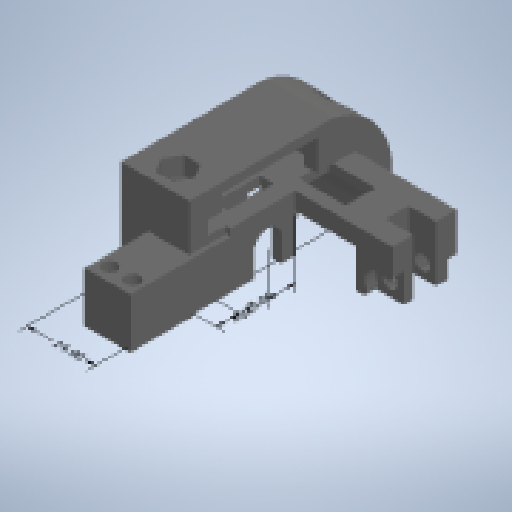
# Autodesk Inventor part: hand_motor_setter_base
Saved by Autodesk Inventor 2024.1 (Build 281209000, 209)
## iProperties
Created: 2025-01-23
Part Number: hand_motor_setter_base
Material: 一般
Document SubType Name: Modeling
Designer: hibik
Density: 1 g/cm^3
Appearance: 既定
Author: hibik
Autodesk Inventor part; units mm, degrees
ref_plane "YZ Plane" through (0, 0, 0) normal (1, 0, 0) x (0, 1, 0)
ref_plane "XZ Plane" through (0, 0, 0) normal (0, 1, 0) x (-1, 0, 0)
sketch "スケッチ1" plane through (0, 0, 0) normal (0, 1, 0) x (-1, 0, 0)
  line L0 (4.5, 6) -> (-4.5, 6) construction
  line L1 (-4.5, 6) -> (-4.5, -18) construction
  line L2 (-4.5, -18) -> (4.5, -18) construction
  line L3 (4.5, -18) -> (4.5, 6) construction
  line L4 (4.5, -6) -> (-4.5, -6)
  line L5 (0, -25.74) -> (0, 13.74) projected
  line L6 (0.5, -18) -> (0.5, -6) construction
  line L7 (4.6, -18.1) -> (-4.6, -18.1)
  line L8 (-4.6, -18.1) -> (-4.6, 6.1)
  line L9 (-4.6, 6.1) -> (4.6, 6.1)
  line L10 (4.6, 6.1) -> (4.6, -18.1)
  line L11 (0.4, -18.1) -> (0.4, -6)
  line L12 (-4.5, -6) -> (-4.6, -6)
  line L13 (4.5, -6) -> (4.6, -6)
  line L14 (6.6, -20.1) -> (-6.6, -20.1)
  line L15 (-6.6, -20.1) -> (-6.6, 8.1)
  line L16 (-6.6, 8.1) -> (6.6, 8.1)
  line L17 (6.6, 8.1) -> (6.6, -20.1)
  line L18 (0.4, -18.1) -> (-14.8, -18.1)
  line L19 (-14.8, -18.1) -> (-14.8, -6)
  line L20 (-14.8, -6) -> (0.4, -6)
  line L21 (0.4, -6) -> (0.4, -18.1)
  line L22 (-6.6, -20.1) -> (-14.8, -20.1)
  line L23 (-14.8, -20.1) -> (-14.8, -18.1)
  point P0 (0, 0)
  point P1 (0, -6)
  point P2 (-6.6, -6)
  point P3 (0, -20.1)
  point P4 (-6.6, -6)
  dimension "d0" = 6
  dimension "d1" = 12
  dimension "d2" = 12
  dimension "d3" = 9
  dimension "d4" = 4
  dimension "d5" = 0.1
  dimension "d6" = 0.1
  dimension "d7" = 0.1
  dimension "d8" = 0.1
  dimension "d9" = 0.1
  dimension "d10" = 2
  dimension "d11" = 2
  dimension "d12" = 15.2
  constraints: 46 end point, 8 parallel, 7 midpoint, 7 perpendicular, 6 horizontal, 4 point on line, 1 collinear, 1 horizontal alignment, 1 vertical alignment, 1 other
  measures "d0" distance from line of L0 point (0, 0)
  measures "d1" distance between parallel lines of L0 L4
  measures "d2" distance between parallel lines of L2 L4
  measures "d3" distance of L1.end L2.end
  measures "d4" distance between parallel lines of L3 L6
  measures "d5" distance between parallel lines of L8 L1
  measures "d6" distance between parallel lines of L10 L3
  measures "d7" distance between parallel lines of L7 L2
  measures "d8" distance between parallel lines of L9 L0
  measures "d9" distance between parallel lines of L11 L6
  measures "d10" distance between parallel lines of L15 L8
  measures "d11" distance between parallel lines of L14 L7
  measures "d12" distance of L19.end L20.end
extrude "押し出し1" add sketch "スケッチ1" against normal blind 2
extrude "押し出し2" add sketch "スケッチ1" against normal blind 12.2 contours L13 L10 L7 L11 L4 | L11 L7 L5 L4 | L10 L9 L5 L16 L17 L14 L7 | L5 L7 L8 L12 L4 | L5 L14 L15 L18 L7 | L9 L8 L20 L15 L16 L5 | L8 L18 L15 L20 | L15 L18 L19 L20 | L22 L23 L18 L15
sketch "スケッチ2" plane through (14.8, 0, -6) normal (1, 0, 0) x (0, 0, -1)
  line L0 (0, 0) -> (0, -12.2) projected
  line L1 (0, -2) -> (14.1, -2)
  line L2 (14.1, 0) -> (14.1, -12.2) projected
  line L3 (0, 0) -> (14.1, 0) projected
  circle A0 centre (6.05, -7.1) radius 6.05
  line L4 (0, 0) -> (0, -12.2) projected
  line L5 (0, 0) -> (14.1, 0) projected
  line L6 (0, 0) -> (0, -12.2) projected
  line L7 (14.1, -12.2) -> (0, -12.2) projected
  line L8 (14.1, 0) -> (14.1, -12.2) projected
  line L9 (12.1, 0) -> (12.1, -12.2)
  point P0 (-6, 0)
  point P1 (14.1, -7.1)
  point P2 (9.3046, -2)
  point P3 (2.7954, -2)
  point P4 (0, -7.1)
  point P5 (2.7954, -12.2)
  point P6 (9.3046, -12.2)
  point P7 (0, -7.1)
  point P8 (12.1, -7.1)
  dimension "d17" = 2
  dimension "d18" = 5.1
  dimension "d21" = 2
  constraints: 4 end point, 4 point on line, 2 tangent, 1 centre point, 1 horizontal, 1 perpendicular
  measures "d17" distance between parallel lines of L3 L1
  measures "d18" distance from line of L1 A0.centre
  measures "d21" distance between parallel lines of L2 L9
extrude "押し出し3" cut sketch "スケッチ2" against normal blind 15.2 contours A0 L7 L0 | A0 L1 L7 | L9 L7 A0
sketch "スケッチ3" plane through (6.6, 0, 8.1) normal (1, 0, 0) x (0, 0, -1)
  circle A0 centre (8.1, -7.1) radius 3
  line L0 (14.1, -12.2) -> (0, -12.2) projected
  line L1 (5.1, -12.2) -> (11.1, -12.2)
  line L2 (11.1, -12.2) -> (11.1, -7.1)
  line L3 (11.1, -7.1) -> (5.1, -7.1)
  line L4 (5.1, -7.1) -> (5.1, -12.2)
  point P0 (8.1, 0)
  dimension "d22" = 6
  dimension "d23" = 7.1
  constraints: 8 end point, 2 parallel, 2 vertical, 1 horizontal, 1 perpendicular, 1 point on line, 1 vertical alignment, 3 other
  measures "d23" distance of point (8.1, 0) point (8.1, -7.1)
extrude "押し出し4" cut sketch "スケッチ3" against normal up to surface (2 mm away)
fillet "フィレット1" radius 0.5 2 edges at (10.7, -7.1, -6) (2.1, -7.1, -6)
sketch "スケッチ4" plane through (-0.4, 0, -6) normal (1, 0, 0) x (0, 0, -1)
  line L0 (-14.1, -12.2) -> (14.1, -12.2) projected
  line L1 (0, -12.2) -> (12.1, -12.2)
  line L2 (12.1, -12.2) -> (12.1, -2)
  line L3 (12.1, -2) -> (0, -2)
  line L4 (0, -2) -> (0, -12.2)
  line L5 (12.1, -7.1) -> (12.1, -12.2) projected
  line L6 (2.7954, -2) -> (9.3046, -2) projected
  point P0 (-6, 0)
  constraints: 8 end point, 2 collinear, 2 parallel, 1 horizontal, 1 midpoint, 1 perpendicular
extrude "押し出し5" cut sketch "スケッチ4" against normal up to surface (4.2 mm away)
ref_plane "作業平面1" through (-3.6, -12.2, 6.1) normal (1, 0, 0) x (0, 0, -1)
sketch "スケッチ5" plane through (-3.6, -12.2, 6.1) normal (1, 0, 0) x (0, 0, -1)
  line L0 (0, 10.2) -> (7.1, 10.2)
  line L1 (7.1, 10.2) -> (7.1, 5.2)
  line L2 (7.1, 5.2) -> (0, 5.2)
  line L3 (0, 5.2) -> (0, 10.2)
  line L4 (9.1, 0) -> (9.1, 5.1) projected
  point P0 (6.1, 12.2)
  dimension "d30" = 5
  dimension "d34" = 2
  constraints: 8 end point, 2 parallel, 1 horizontal, 1 perpendicular
  measures "d30" distance of L0.end L1.end
  measures "d34" distance between parallel lines of L1 L4
extrude "押し出し6" add sketch "スケッチ5" along normal blind 1.5
fillet "フィレット2" radius 3 2 edges at (-2.85, -7, -1) (-2.85, -7, 6.1)
sketch "スケッチ6" plane through (0, 0, 0) normal (0, 1, 0) x (1, 0, 0)
  line L0 (-6.6, -8.1) -> (6.6, -8.1) projected
  line L1 (5.6, -8.1) -> (2.6, -8.1)
  line L2 (2.6, -8.1) -> (2.6, -0.1)
  line L3 (2.6, -0.1) -> (5.6, -0.1)
  line L4 (5.6, -0.1) -> (5.6, -8.1)
  line L5 (6.6, -8.1) -> (6.6, 6) projected
  line L6 (-9.3, -8.1) -> (-7.3, -8.1)
  line L7 (-7.3, -8.1) -> (-7.3, 13.8)
  line L8 (-7.3, 13.8) -> (-9.3, 13.8)
  line L9 (-9.3, 13.8) -> (-9.3, -8.1)
  line L10 (-4.6, -6.1) -> (4.6, -6.1) projected
  line L11 (-7.3, -8.1) -> (2.6, -8.1)
  line L12 (2.6, -8.1) -> (2.6, -6.1)
  line L13 (2.6, -6.1) -> (-7.3, -6.1)
  line L14 (-7.3, -6.1) -> (-7.3, -8.1)
  line L15 (-9.3, 13.8) -> (2.9, 13.8)
  line L16 (2.9, 13.8) -> (2.9, 15.8)
  line L17 (2.9, 15.8) -> (-9.3, 15.8)
  line L18 (-9.3, 15.8) -> (-9.3, 13.8)
  line L19 (-9.3, 12.3) -> (-7.3, 12.3)
  line L20 (-9.3, -4.6) -> (-7.3, -4.6)
  line L21 (-7.3, -1.4667) -> (-9.3, -1.4667)
  line L22 (-9.3, -1.4667) -> (-9.3, 1.5333)
  line L23 (-9.3, 1.5333) -> (-7.3, 1.5333)
  line L24 (-7.3, 1.5333) -> (-7.3, -1.4667)
  line L25 (-7.3, 6.1667) -> (-9.3, 6.1667)
  line L26 (-9.3, 6.1667) -> (-9.3, 9.1667)
  line L27 (-9.3, 9.1667) -> (-7.3, 9.1667)
  line L28 (-7.3, 9.1667) -> (-7.3, 6.1667)
  circle A0 centre (-4.5, 8.6) radius 1
  circle A1 centre (-4.5, -0.9) radius 1
  line L29 (-9.3, 3.85) -> (-0.8107, 3.85)
  line L30 (2.9, 15.8) -> (-9.3, 15.8)
  line L31 (-9.3, 15.8) -> (-9.3, 20.1)
  line L32 (-9.3, 20.1) -> (2.9, 20.1)
  line L33 (2.9, 20.1) -> (2.9, 15.8)
  line L34 (14.8, 20.1) -> (-6.6, 20.1) projected
  point P0 (0, 0)
  point P1 (-9.3, 6.1667)
  point P2 (-7.3, 3.85)
  point P3 (2.6, -8.1)
  point P4 (2.6, -8.1)
  dimension "d35" = 4
  dimension "d36" = 8
  dimension "d37" = 3
  dimension "d40" = 9.9
  dimension "d41" = 2
  dimension "d42" = 19.9
  dimension "d43" = 2
  dimension "d44" = 10.2
  dimension "d45" = 1.5
  dimension "d46" = 1.5
  dimension "d53" = 3
  dimension "d54" = 3
  dimension "d55" = 4.6333
  dimension "d56" = 4.6333
  dimension "d57" = 4.6333
  dimension "d60" = 2
  dimension "d61" = 2
  dimension "d62" = 7.1
  dimension "d63" = 9.5
  constraints: 62 end point, 14 parallel, 12 point on line, 9 perpendicular, 8 horizontal, 3 collinear, 2 centre point, 1 symmetric about line, 1 vertical alignment, 1 other
  measures "d35" distance between parallel lines of L5 L2
  measures "d36" distance of L3.end L1.start
  measures "d37" distance between parallel lines of L4 L2
  measures "d40" distance between parallel lines of L2 L7
  measures "d41" distance of L6.start L6.end
  measures "d42" distance between parallel lines of L8 L13
  measures "d43" distance of L17.end L8.end
  measures "d44" distance between parallel lines of L16 L7
  measures "d45" distance between parallel lines of L15 L19
  measures "d46" distance between parallel lines of L13 L20
  measures "d53" distance between parallel lines of L21 L23
  measures "d54" distance between parallel lines of L27 L25
  measures "d55" distance between parallel lines of L13 L21
  measures "d56" distance between parallel lines of L25 L23
  measures "d57" distance between parallel lines of L15 L27
  measures "d60" diameter of A0
  measures "d61" diameter of A1
  measures "d62" distance from line of L2 A1.centre
  measures "d63" distance of A1.centre A0.centre
extrude "押し出し7" add sketch "スケッチ6" along normal blind 6.6 contours L11 L7 L13 L10 L2 L0 | L2 L3 L4 L0 | L6 L9 L20 L7 | L9 L23 L7 L21 | L9 L27 L7 L25 | L9 L8 L7 L19 | L18 L17 L16 L15 L8 | L31 L32 L33 L17 | A0 | A1
chamfer "面取り1" distance 6 distance2 2 1 edges at (5.6, 3.3, 0.1) measured on face at (5.6, 2.2, 5.4333)
sketch "スケッチ7" plane through (-6.6, -12.2, -20.1) normal (-1, 0, 0) x (0, 0, 1)
  line L0 (0, 12.2) -> (0, 0) projected
  line L1 (28.2, 0) -> (0, 0) projected
  line L2 (28.2, 12.2) -> (28.2, 0) projected
  line L3 (26.2, 12.2) -> (28.2, 12.2) projected
  line L4 (6.3, 12.2) -> (26.2, 12.2) projected
  line L5 (0, 12.2) -> (6.3, 12.2) projected
  point P0 (20.1, 12.2)
extrude "押し出し8" add sketch "スケッチ7" along normal up to surface (2.7 mm away)
sketch "スケッチ8" plane through (0, 6.6, 0) normal (0, 1, 0) x (1, 0, 0)
  line L0 (14.8, 20.1) -> (-9.3, 20.1) projected
  line L1 (-9.3, -8.1) -> (5.6, -8.1)
  line L2 (5.6, -8.1) -> (5.6, 20.1)
  line L3 (5.6, 20.1) -> (-9.3, 20.1)
  line L4 (-9.3, 20.1) -> (-9.3, -8.1)
  line L5 (5.6, -8.1) -> (5.6, -6.1) projected
  circle A0 centre (-1.85, 23.1) radius 1.6
  circle A1 centre (-1.85, -11.1) radius 1.6
  line L6 (5.6, 6) -> (-9.3, 6)
  line L7 (-9.3, -8.1) -> (5.6, -8.1)
  line L8 (5.6, -8.1) -> (5.6, -16.1)
  line L9 (5.6, -16.1) -> (-9.3, -16.1)
  line L10 (-9.3, -16.1) -> (-9.3, -8.1)
  line L11 (-9.3, 20.1) -> (5.6, 20.1)
  line L12 (5.6, 20.1) -> (5.6, 28.1)
  line L13 (5.6, 28.1) -> (-9.3, 28.1)
  line L14 (-9.3, 28.1) -> (-9.3, 20.1)
  line L15 (-9.3, 20.1) -> (-9.3, -8.1) projected
  line L16 (-9.3, -8.1) -> (5.6, -8.1) projected
  point P0 (0, 0)
  point P1 (-1.85, 20.1)
  dimension "d64" = 3.2
  dimension "d65" = 3.2
  dimension "d66" = 3
  dimension "d67" = 8
  constraints: 26 end point, 6 parallel, 5 collinear, 3 horizontal, 3 midpoint, 3 perpendicular, 2 centre point, 2 vertical alignment, 1 point on line, 1 symmetric about line, 1 other
  measures "d64" diameter of A0
  measures "d65" diameter of A1
  measures "d66" distance from line of A0.centre L0
  measures "d67" distance of L13.end L3.end
extrude "押し出し9" add sketch "スケッチ8" along normal blind 2
extrude "押し出し10" add sketch "スケッチ8" against normal up to surface (18.8 mm away) contours L0 L14 L13 L12 | L1 L8 L9 L10
sketch "スケッチ9" plane through (0, 8.6, 0) normal (0, 1, 0) x (1, 0, 0)
  circle A0 centre (-1.85, -11.1) radius 1.6 projected
  circle A1 centre (-1.85, 23.1) radius 1.6 projected
  line L0 (1.4409, -11.1) -> (-0.2046, -13.95)
  line L1 (-0.2046, -13.95) -> (-3.4954, -13.95)
  line L2 (-3.4954, -13.95) -> (-5.1409, -11.1)
  line L3 (-5.1409, -11.1) -> (-3.4954, -8.25)
  line L4 (-3.4954, -8.25) -> (-0.2046, -8.25)
  line L5 (-0.2046, -8.25) -> (1.4409, -11.1)
  line L6 (-0.2046, 25.95) -> (1.4409, 23.1)
  line L7 (1.4409, 23.1) -> (-0.2046, 20.25)
  line L8 (-0.2046, 20.25) -> (-3.4954, 20.25)
  line L9 (-3.4954, 20.25) -> (-5.1409, 23.1)
  line L10 (-5.1409, 23.1) -> (-3.4954, 25.95)
  line L11 (-3.4954, 25.95) -> (-0.2046, 25.95)
  point P0 (0, 0)
  dimension "d72" = 5.7
  constraints: 24 end point, 2 coincident, 2 horizontal, 1 parallel, 26 other
  measures "d72" distance between parallel lines of L1 L4
extrude "押し出し11" cut sketch "スケッチ9" against normal blind 6.5 contours A0 | A1 | L0 L1 L2 L3 L4 L5 | L6 L7 L8 L9 L10 L11
sketch "スケッチ10" plane through (0, 8.6, 0) normal (0, 1, 0) x (1, 0, 0)
  circle A0 centre (-1.85, -11.1) radius 1.6 projected
  circle A1 centre (-1.85, 23.1) radius 1.6 projected
  line L0 (-3.6398, -8) -> (-0.0602, -8)
  line L1 (-0.0602, -8) -> (1.7296, -11.1)
  line L2 (1.7296, -11.1) -> (-0.0602, -14.2)
  line L3 (-0.0602, -14.2) -> (-3.6398, -14.2)
  line L4 (-3.6398, -14.2) -> (-5.4296, -11.1)
  line L5 (-5.4296, -11.1) -> (-3.6398, -8)
  line L6 (-3.6398, 26.2) -> (-0.0602, 26.2)
  line L7 (-0.0602, 26.2) -> (1.7296, 23.1)
  line L8 (1.7296, 23.1) -> (-0.0602, 20)
  line L9 (-0.0602, 20) -> (-3.6398, 20)
  line L10 (-3.6398, 20) -> (-5.4296, 23.1)
  line L11 (-5.4296, 23.1) -> (-3.6398, 26.2)
  line L12 (-0.2046, -13.95) -> (-3.4954, -13.95) projected
  line L13 (-0.2046, 20.25) -> (-3.4954, 20.25) projected
  point P0 (0, 0)
  dimension "d75" = 6.2
  constraints: 24 end point, 2 coincident, 2 parallel, 1 equal length, 26 other
  measures "d75" distance between parallel lines of L0 L3
extrude "押し出し12" cut sketch "スケッチ10" against normal blind 4 contours A0 | A1 | L0 L1 L2 L3 L4 L5 | L6 L7 L8 L9 L10 L11
sketch "スケッチ11" plane through (14.8, 0, -6) normal (1, 0, 0) x (0, 0, -1)
  arc A0 (0, -3.6215) -> (0.9237, -3.887) centre (0.5, -3.6215) ccw projected
  arc A1 (2.7954, -2) -> (0.9237, -3.887) centre (6.05, -7.1) ccw projected
  line L0 (2.7954, -2) -> (9.3046, -2) projected
  arc A2 (12.1, -7.1) -> (9.3046, -2) centre (6.05, -7.1) ccw projected
  line L1 (12.1, -7.1) -> (12.1, -12.2) projected
  line L2 (14.1, -12.2) -> (12.1, -12.2) projected
  line L3 (14.1, 0) -> (14.1, -12.2) projected
  line L4 (0, 0) -> (14.1, 0) projected
  line L5 (0, 0) -> (0, -3.6215) projected
  line L6 (9.3046, -2) -> (14.1, -2)
  point P0 (-6, 0)
  constraints: 2 end point, 1 perpendicular, 1 point on line
extrude "押し出し13" add sketch "スケッチ11" along normal blind 5 contours L5 L4 L3 L6 L0 A1 A0
sketch "スケッチ12" plane through (19.8, 0, -6) normal (1, 0, 0) x (0, 0, -1)
  line L0 (0, -7.1) -> (0, -12.2) projected
  line L1 (14.1, 0) -> (0, 0) projected
  line L2 (14.1, -2) -> (14.1, -12.2) projected
  line L3 (14.1, -12.2) -> (0, -12.2)
  line L4 (0, -12.2) -> (0, 0)
  line L5 (0, 0) -> (14.1, 0)
  line L6 (14.1, 0) -> (14.1, -12.2)
  point P0 (-6, 0)
  constraints: 8 end point, 2 parallel, 1 horizontal, 1 perpendicular
extrude "押し出し14" add sketch "スケッチ12" along normal blind 2
sketch "スケッチ13" plane through (14.8, -12.2, -20.1) normal (0, 0, -1) x (-1, 0, 0)
  line L0 (8.2, 12.2) -> (-7, 12.2) projected
  line L1 (-7, 12.2) -> (-13, 12.2)
  line L2 (-13, 12.2) -> (-13, 0)
  line L3 (-13, 0) -> (-7, 0)
  line L4 (-7, 0) -> (-7, 12.2)
  circle A0 centre (-10, 3) radius 1.6
  line L5 (-5, 0) -> (-7, 0) projected
  point P0 (14.8, 12.2)
  dimension "d98" = 3.2
  dimension "d99" = 3
  dimension "d100" = 3
  dimension "d101" = 6
  constraints: 8 end point, 2 parallel, 1 centre point, 1 collinear, 1 horizontal, 1 perpendicular
  measures "d98" diameter of A0
  measures "d99" distance from line of L3 A0.centre
  measures "d100" distance from line of L2 A0.centre
  measures "d101" distance of L0.end L1.end
extrude "押し出し15" add sketch "スケッチ13" against normal up to surface (14.1 mm away)
sketch "スケッチ14" plane through (19.8, -12.2, -20.1) normal (0, -1, 0) x (1, 0, 0)
  line L0 (8, 0) -> (8, 14.1) projected
  line L1 (8, 4.55) -> (2, 4.55)
  line L2 (2, 4.55) -> (2, 9.55)
  line L3 (2, 9.55) -> (8, 9.55)
  line L4 (8, 9.55) -> (8, 4.55)
  line L5 (0, 14.1) -> (0, 0) projected
  point P0 (-19.8, 20.1)
  point P1 (2, 7.05)
  point P2 (0, 7.05)
  point P3 (8, 9.55)
  dimension "d104" = 2
  dimension "d105" = 5
  constraints: 8 end point, 2 midpoint, 2 parallel, 1 horizontal, 1 horizontal alignment, 1 perpendicular, 1 point on line
  measures "d104" distance between parallel lines of L5 L2
  measures "d105" distance of L1.end L2.end
extrude "押し出し16" cut sketch "スケッチ14" against normal through all
sketch "スケッチ15" plane through (14.8, -12.2, -20.1) normal (0, 0, -1) x (-1, 0, 0)
  circle A0 centre (-10, 3) radius 1.6 projected
  line L0 (-11.7321, 0) -> (-13.4641, 3)
  line L1 (-13.4641, 3) -> (-11.7321, 6)
  line L2 (-11.7321, 6) -> (-8.2679, 6)
  line L3 (-8.2679, 6) -> (-6.5359, 3)
  line L4 (-6.5359, 3) -> (-8.2679, 0)
  line L5 (-8.2679, 0) -> (-11.7321, 0)
  line L6 (-5, 0) -> (-13, 0) projected
  line L7 (-13, 12.2) -> (-13, 0) projected
  point P0 (14.8, 12.2)
  point P1 (-13, 3.8038)
  point P2 (-11.7321, 0)
  constraints: 12 end point, 1 coincident, 1 collinear, 1 horizontal, 13 other
extrude "押し出し17" cut sketch "スケッチ15" against normal blind 2 contours A0 | L6 L7 L0 | L0 L7 L1 L2 L3 L4 L5
sketch "スケッチ16" plane through (6.6, -3.6215, -6) normal (0, 0, 1) x (1, 0, 0)
  circle A0 centre (18.2, -5.5785) radius 1.6 projected
  circle A1 centre (18.2, -5.5785) radius 3
  circle A2 centre (18.2, -5.5785) radius 1.6 projected
  line L0 (13.2, 0) -> (0, 0) projected
  line L1 (13.2, 0) -> (13.2, -8.5785) projected
  line L2 (13.2, -8.5785) -> (21.2, -8.5785) projected
  line L3 (21.2, 3.6215) -> (21.2, -8.5785) projected
  line L4 (0, 3.6215) -> (21.2, 3.6215) projected
  line L5 (0, 3.6215) -> (0, 0) projected
  point P0 (-6.6, 3.6215)
  point P1 (21.2, -5.5785)
  point P2 (18.2, -8.5785)
  constraints: 1 centre point, 1 coincident, 1 tangent
extrude "押し出し18" cut sketch "スケッチ16" against normal blind 2.5 contours A1 | L3 L2 A1
fillet "フィレット3" radius 1 2 edges at (24.8, -12.2, -7.25) (27.8, -9.2, -7.25)
sketch "スケッチ17" plane through (0, 0, 0) normal (0, 1, 0) x (1, 0, 0)
  circle A0 centre (-4.5, 8.6) radius 1 projected
  circle A1 centre (-4.5, -0.9) radius 1 projected
  line L0 (27.8, 10.55) -> (21.8, 10.55) projected
  line L1 (21.8, 10.55) -> (21.8, 15.55) projected
  line L2 (21.8, 15.55) -> (27.8, 15.55) projected
  line L3 (27.8, 20.1) -> (27.8, 15.55) projected
  line L4 (27.8, 20.1) -> (5.6, 20.1) projected
  line L5 (5.6, 20.1) -> (2.9, 20.1) projected
  line L6 (-7.3, 13.8) -> (2.9, 13.8) projected
  line L7 (-7.3, 12.3) -> (-7.3, 13.8) projected
  line L8 (-7.3, -6.1) -> (2.6, -6.1) projected
  line L9 (2.6, -6.1) -> (2.6, -0.1) projected
  line L10 (2.6, -0.1) -> (3.6, -0.1) projected
  line L11 (5.6, -6.1) -> (3.6, -0.1) projected
  line L12 (5.6, -6.1) -> (5.6, -8.1) projected
  line L13 (5.6, -8.1) -> (6.6, -8.1) projected
  line L14 (6.6, -8.1) -> (6.6, 6) projected
  line L15 (6.6, 6) -> (27.8, 6) projected
  line L16 (27.8, 10.55) -> (27.8, 6) projected
  line L17 (2.6, -6.1) -> (2.6, -0.1) projected
  line L18 (2.6, -0.1) -> (6.6, -0.1)
  line L19 (6.6, -0.1) -> (6.6, -12.1)
  line L20 (6.6, -12.1) -> (2.6, -12.1)
  line L21 (2.6, -12.1) -> (2.6, -0.1)
  line L22 (6.6, -8.1) -> (6.6, 6) projected
  line L23 (2.9, 20.1) -> (2.9, 13.8) projected
  line L24 (-9.3, 12.3) -> (-7.3, 12.3) projected
  line L25 (-9.3, 12.3) -> (-9.3, 9.1667) projected
  line L26 (-7.3, 9.1667) -> (-9.3, 9.1667) projected
  line L27 (-7.3, 6.1667) -> (-7.3, 9.1667) projected
  line L28 (-9.3, 6.1667) -> (-7.3, 6.1667) projected
  line L29 (-9.3, 6.1667) -> (-9.3, 1.5333) projected
  line L30 (-7.3, 1.5333) -> (-9.3, 1.5333) projected
  line L31 (-7.3, -1.4667) -> (-7.3, 1.5333) projected
  line L32 (-9.3, -1.4667) -> (-7.3, -1.4667) projected
  line L33 (-9.3, -1.4667) -> (-9.3, -4.6) projected
  line L34 (-7.3, -4.6) -> (-9.3, -4.6) projected
  line L35 (-7.3, -6.1) -> (-7.3, -4.6) projected
  point P0 (0, 0)
  dimension "d116" = 12
  constraints: 8 end point, 2 parallel, 1 collinear, 1 horizontal, 1 perpendicular
  measures "d116" distance of L18.end L19.end
extrude "押し出し19" cut sketch "スケッチ17" along normal up to surface (6.6 mm away) contours L14 L13 L12 L11 L18 | L19 L20 L21 L9 L10 L11 L12 L13
sketch "スケッチ18" plane through (0, 0, 0) normal (0, 1, 0) x (1, 0, 0)
  line L0 (2.9, 11.8) -> (5.6, 11.8)
  line L1 (5.6, 11.8) -> (5.6, 20.1)
  line L2 (5.6, 20.1) -> (2.9, 20.1)
  line L3 (2.9, 20.1) -> (2.9, 11.8)
  line L4 (5.6, 20.1) -> (2.9, 20.1) projected
  line L5 (5.6, -12.1) -> (5.6, 20.1) projected
  line L6 (2.9, 20.1) -> (2.9, 13.8) projected
  line L7 (-7.3, 13.8) -> (2.9, 13.8) projected
  point P0 (0, 0)
  dimension "d122" = 2
  constraints: 8 end point, 3 collinear, 2 parallel, 1 horizontal, 1 perpendicular
  measures "d122" distance between parallel lines of L7 L0
extrude "押し出し20" add sketch "スケッチ18" along normal up to surface (6.6 mm away)
sketch "スケッチ23" plane through (6.6, 0, 8.1) normal (1, 0, 0) x (0, 0, -1)
  line L0 (11.1, -7.1) -> (11.1, -12.2) projected
  line L1 (14.1, -12.2) -> (11.1, -12.2) projected
  line L2 (14.1, -7.1) -> (14.1, -12.2) projected
  arc A0 (15.0237, -3.887) -> (14.1, -7.1) centre (20.15, -7.1) ccw projected
  arc A1 (14.1, -3.6215) -> (15.0237, -3.887) centre (14.6, -3.6215) ccw projected
  line L3 (14.1, 0) -> (14.1, -3.6215) projected
  line L4 (0, 0) -> (14.1, 0) projected
  line L5 (0, 0) -> (0, -12.2) projected
  line L6 (5.1, -12.2) -> (0, -12.2) projected
  line L7 (5.1, -12.2) -> (5.1, -7.1) projected
  arc A2 (11.1, -7.1) -> (5.1, -7.1) centre (8.1, -7.1) ccw projected
  arc A3 (11.1, -7.1) -> (5.1, -7.1) centre (8.1, -7.1) ccw projected
  circle A4 centre (8.1, -7.1) radius 5.5
  line L8 (8.1, -1.6) -> (-21.9, -1.6)
  line L9 (-21.9, -1.6) -> (-21.9, -12.6)
  line L10 (-21.9, -12.6) -> (8.1, -12.6)
  line L11 (8.1, -12.6) -> (8.1, -1.6)
  line L12 (-8, 8.6) -> (-8, -12.2) projected
  line L13 (-8, -12.2) -> (-8, -12.6)
  line L14 (11.1, -12.2) -> (11.1, -7.1) projected
  arc A5 (11.1, -7.1) -> (5.1, -7.1) centre (8.1, -7.1) ccw projected
  line L15 (5.1, -7.1) -> (5.1, -12.2) projected
  line L16 (2, -12.2) -> (5.1, -12.2) projected
  line L17 (2, -2) -> (2, -12.2) projected
  line L18 (14.1, -2) -> (2, -2) projected
  line L19 (14.1, -2) -> (14.1, -3.6215) projected
  arc A6 (14.1, -3.6215) -> (15.0237, -3.887) centre (14.6, -3.6215) ccw projected
  arc A7 (15.0237, -3.887) -> (14.1, -7.1) centre (20.15, -7.1) ccw projected
  line L20 (14.1, -7.1) -> (14.1, -12.2) projected
  line L21 (11.1, -12.2) -> (14.1, -12.2) projected
  line L22 (2, -2) -> (2, -12.2) projected
  line L23 (2, -12.2) -> (2, -12.6)
  line L24 (2, -2) -> (2, -1.6)
  line L25 (-8, -12.2) -> (0, -12.2) projected
  point P0 (8.1, 0)
  dimension "d138" = 11
  dimension "d139" = 30
  constraints: 14 end point, 3 horizontal, 3 perpendicular, 3 point on line, 2 parallel, 1 coincident, 1 collinear, 1 vertical alignment, 2 other
  measures "d139" distance of L9.end L10.end
extrude "押し出し24" add sketch "スケッチ23" against normal blind 10 contours L10 L9 L8 L12 L13 | L6 L5 L8 L24 L17 | L12 L8 L5 L25
sketch "スケッチ24" plane through (0, -2, 0) normal (0, -1, 0) x (1, 0, 0)
  line L0 (2.9, 5.1) -> (-0.1, 5.1)
  line L1 (-0.1, 5.1) -> (-0.1, -5)
  line L2 (-0.1, -5) -> (2.9, -5)
  line L3 (4.6, -3) -> (4.6, 3) projected
  line L4 (-4.6, 6.1) -> (4.6, 6.1) projected
  line L5 (4.6, -6) -> (-0.4, -6) projected
  line L6 (-2.1, 2) -> (-2.1, -1) projected
  line L7 (-2.1, 6.1) -> (-2.1, -1) projected
  line L8 (-2.1, -1) -> (-3.6, -1) projected
  line L9 (-3.6, -1) -> (-3.6, 6.1) projected
  line L10 (-3.6, 6.1) -> (-4.6, 6.1) projected
  line L11 (-4.6, 6.1) -> (-4.6, -18.1) projected
  line L12 (-0.4, -18.1) -> (-4.6, -18.1) projected
  line L13 (-0.4, -18.1) -> (-0.4, -15.3046) projected
  line L14 (14.8, -15.3046) -> (-0.4, -15.3046) projected
  line L15 (14.8, -20.1) -> (14.8, -15.3046) projected
  line L16 (14.8, -20.1) -> (19.8, -20.1) projected
  line L17 (19.8, -8.7954) -> (19.8, -20.1) projected
  line L18 (19.8, -8.7954) -> (-0.4, -8.7954) projected
  line L19 (-0.4, -8.7954) -> (-0.4, -6) projected
  line L20 (-0.4, -6) -> (4.6, -6) projected
  line L21 (4.6, -6) -> (4.6, 6.1) projected
  line L22 (4.6, 6.1) -> (-2.1, 6.1) projected
  line L23 (14.8, -15.3046) -> (4.6, -15.3046)
  line L24 (4.6, -15.3046) -> (4.6, -8.7954)
  line L25 (4.6, -8.7954) -> (14.8, -8.7954)
  line L26 (14.8, -8.7954) -> (14.8, -15.3046)
  line L27 (4.6, -3) -> (4.6, -6) projected
  line L28 (2.9, 5.1) -> (2.9, -5)
  point P0 (0, 0)
  dimension "d143" = 1
  dimension "d144" = 1
  dimension "d145" = 2
  dimension "d146" = 3
  constraints: 16 end point, 3 parallel, 2 horizontal, 2 perpendicular, 1 collinear, 1 point on line, 1 vertical
  measures "d143" distance between parallel lines of L4 L0
  measures "d144" distance between parallel lines of L5 L2
  measures "d145" distance between parallel lines of L6 L1
  measures "d146" distance of L1.end L2.end
extrude "押し出し25" cut sketch "スケッチ24" against normal up to surface (2 mm away) contours L28 L2 L1 L0 | L18 L26 L14 L24
sketch "スケッチ26" plane through (0, -12.2, 0) normal (0, -1, 0) x (1, 0, 0)
  arc A0 (-3.4, 10.7031) -> (-3.4, 11.4969) centre (-1.85, 11.1) ccw projected
  circle A1 centre (-1.85, 11.1) radius 1.6
  point P0 (0, 0)
  constraints: 1 centre point, 1 coincident, 1 concentric
extrude "押し出し27" cut sketch "スケッチ26" against normal through all
sketch "スケッチ27" plane through (6.6, -1.6, 30) normal (0, 1, 0) x (1, 0, 0)
  circle A0 centre (-2.5, 3) radius 1.6
  circle A1 centre (-7.5, 3) radius 1.6
  line L0 (-10, 0) -> (-10, 13.9) projected
  line L1 (0, 21.9) -> (0, 0) projected
  line L2 (0, 0) -> (-10, 0) projected
  point P0 (-6.6, 30)
  dimension "d155" = 3.2
  dimension "d156" = 3.2
  dimension "d157" = 2.5
  dimension "d158" = 2.5
  dimension "d159" = 3
  constraints: 2 centre point, 1 horizontal alignment
  measures "d155" diameter of A0
  measures "d156" diameter of A1
  measures "d157" distance from line of L0 A1.centre
  measures "d158" distance from line of L1 A0.centre
  measures "d159" distance from line of L2 A1.centre
extrude "押し出し28" cut sketch "スケッチ27" against normal through all
sketch "スケッチ29" plane through (-9.3, -12.2, 16.1) normal (-1, 0, 0) x (0, 0, 1)
  arc A0 (-31.4046, 10.2) -> (-34.2, 5.1) centre (-28.15, 5.1) ccw projected
  circle A1 centre (-28.15, 5.1) radius 5
  point P0 (-16.1, 12.2)
  dimension "d163" = 10
  constraints: 1 centre point, 1 coincident
  measures "d163" diameter of A1
extrude "押し出し29" cut sketch "スケッチ29" against normal up to surface (4.7 mm away)
sketch "スケッチ30" plane through (5.6, -12.2, -20.1) normal (1, 0, 0) x (0, 0, -1)
  arc A0 (-2, 5.1) -> (-4.7954, 10.2) centre (-8.05, 5.1) ccw projected
  circle A1 centre (-8.05, 5.1) radius 5 projected
  circle A2 centre (-8.05, 5.1) radius 16.05
  line L0 (8, 0) -> (8, 20.8) projected
  line L1 (8, 0) -> (8, 20.8) projected
  line L2 (-0.1, 20.8) -> (3, 20.8) projected
  line L3 (3, 20.8) -> (6.1, 20.8) projected
  line L4 (6.1, 20.8) -> (3, 20.8) projected
  line L5 (3, 20.8) -> (-0.1, 20.8) projected
  line L6 (-34.3, 20.8) -> (-31.2, 20.8) projected
  line L7 (-31.2, 20.8) -> (-28.1, 20.8) projected
  line L8 (-28.1, 20.8) -> (-31.2, 20.8) projected
  line L9 (-31.2, 20.8) -> (-34.3, 20.8) projected
  line L10 (-36.2, 20.8) -> (8, 20.8) projected
  line L11 (8, 20.8) -> (-36.2, 20.8) projected
  line L12 (-32.8, 0) -> (-29.6, 0) projected
  line L13 (1.4, 0) -> (4.6, 0) projected
  line L14 (-26.2, 0) -> (-23.1, 0) projected
  line L15 (-23.1, 0) -> (-36.2, 0) projected
  line L16 (8, 0) -> (-36.2, 0) projected
  line L17 (0, 0) -> (8, 0) projected
  line L18 (0, 0) -> (-2, 0) projected
  line L19 (-2, 0) -> (-26.2, 0) projected
  point P0 (-20.1, 12.2)
  point P1 (7.1682, 0)
  point P2 (8, 5.1)
  point P3 (-4.7165, 20.8)
  constraints: 1 centre point, 1 coincident, 1 tangent
extrude "押し出し30" cut sketch "スケッチ30" against normal through all contours L0 L16 A2 | A2 L10 L2 L3 L0
sketch "スケッチ32" plane through (-9.3, -12.2, 16.1) normal (-1, 0, 0) x (0, 0, 1)
  arc A0 (-31.4835, 20.8) -> (-43.3682, 0) centre (-28.15, 5.1) ccw projected
  line L0 (-43.3682, 0) -> (0, 0) projected
  line L1 (0, 0) -> (0, 20.8) projected
  line L2 (-31.4835, 20.8) -> (0, 20.8) projected
  circle A1 centre (-28.15, 5.1) radius 5 projected
  line L3 (-17.6333, 12.2) -> (-17.6333, 18.8) projected
  line L4 (-22.2667, 12.2) -> (-17.6333, 12.2) projected
  line L5 (-22.2667, 12.2) -> (-22.2667, 18.8) projected
  line L6 (-22.2667, 18.8) -> (-17.6333, 18.8) projected
  line L7 (-25.2667, 12.2) -> (-25.2667, 18.8) projected
  line L8 (-28.4, 12.2) -> (-25.2667, 12.2) projected
  line L9 (-28.4, 12.2) -> (-28.4, 18.8) projected
  line L10 (-28.4, 18.8) -> (-25.2667, 18.8) projected
  line L11 (-14.6333, 18.8) -> (-11.5, 18.8) projected
  line L12 (-11.5, 12.2) -> (-11.5, 18.8) projected
  line L13 (-14.6333, 12.2) -> (-11.5, 12.2) projected
  line L14 (-14.6333, 12.2) -> (-14.6333, 18.8) projected
  line L15 (0, 20.8) -> (-7, 20.8)
  line L16 (-7, 20.8) -> (-7, 0)
  line L17 (-7, 0) -> (0, 0)
  line L18 (0, 0) -> (0, 20.8)
  point P0 (-16.1, 12.2)
  point P1 (-7, 20.8)
  dimension "d172" = 7
  constraints: 8 end point, 2 parallel, 1 horizontal, 1 perpendicular, 1 point on line
  measures "d172" distance between parallel lines of L1 L16
extrude "押し出し32" add sketch "スケッチ32" along normal blind 2 contours L2 L1 L0 L16
sketch "スケッチ33" plane through (-3.4, -1.6, 16.1) normal (0, 0, 1) x (1, 0, 0)
  circle A0 centre (-4.9, 7.2) radius 3
  circle A1 centre (-4.9, 7.2) radius 1.35
  line L0 (9, 10.2) -> (-7.9, 10.2) projected
  line L1 (-7.9, -10.6) -> (-7.9, 10.2) projected
  point P0 (3.4, 1.6)
  dimension "d175" = 2.7
  dimension "d176" = 6
  constraints: 2 centre point, 2 tangent, 1 coincident
  measures "d175" diameter of A1
  measures "d176" diameter of A0
extrude "押し出し33" cut sketch "スケッチ33" against normal up to surface (7 mm away) contours A1
chamfer "面取り2" distance 2 angle 45 1 edges at (-11.3, -1.8, 9.1)
equation "\"d21\" = d17"
equation "\"d54\" = d53"
equation "\"d55\" = d57"
equation "\"d56\" = d57"
equation "\"d158\" = d157"
